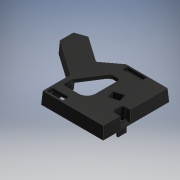
# Autodesk Inventor part: black_plastic_cover
Saved by Autodesk Inventor 2018 (Build 220112000, 112)
## iProperties
Created: 2019-03-10
Part Number: black_plastic_cover
Material: Generic
Document SubType Name: Modeling
Designer: ZEUSLAP
Density: 1 g/cm^3
Appearance: Default
Author: ZEUSLAP
Autodesk Inventor part; units mm, degrees
ref_plane "YZ Plane" through (0, 0, 0) normal (1, 0, 0) x (0, 1, 0)
ref_plane "XZ Plane" through (0, 0, 0) normal (0, 1, 0) x (-1, 0, 0)
ref_plane "XY Plane" through (0, 0, 0) normal (0, 0, 1) x (1, 0, 0)
sketch "Sketch1" plane through (0, 0, 0) normal (0, 0, 1) x (1, 0, 0)
  line L0 (18.3537, -19.4997) -> (-18.1463, -19.4997)
  line L1 (-18.2567, 19.3967) -> (18.3537, -19.4997) construction
  line L2 (18.1463, 19.4997) -> (-18.1463, -19.4997) construction
  line L3 (18.1463, 19.4997) -> (-6.8537, 19.4997) construction
  line L4 (-18.1463, -19.4997) -> (-18.1463, -2.9997) construction
  line L5 (18.1463, 19.4997) -> (-16.8537, 19.4997) construction
  line L6 (-16.8537, 19.4997) -> (-16.8537, 11.9997) construction
  line L7 (-6.8537, 19.4997) -> (-16.8537, 11.9997)
  line L8 (-38.8537, 19.4997) -> (-32.3537, 19.4997) construction
  line L9 (-16.8537, 11.9997) -> (-31.3344, 22.1392)
  line L10 (-31.3344, 22.1392) -> (-38.8537, 19.4997)
  line L11 (-38.8537, 19.4997) -> (-38.8537, 11.4997)
  line L12 (-38.8537, 11.4997) -> (-18.1463, -2.9997)
  line L13 (-18.1463, -19.4997) -> (-18.1463, -2.9997)
  line L14 (18.1463, 19.4997) -> (-6.8537, 19.4997) construction
  line L15 (-16.8537, 19.4997) -> (-38.8537, 19.4997) construction
  line L16 (-6.8537, 19.4997) -> (18.1463, 19.4997)
  line L17 (18.3537, -19.4997) -> (18.3537, -8.4997) construction
  line L18 (18.3537, -8.4997) -> (12.8537, -8.4997)
  line L19 (12.8537, -8.4997) -> (12.8537, -3.504)
  line L20 (12.8537, -3.504) -> (18.1463, -3.504)
  line L21 (18.1463, 19.4997) -> (18.1463, -3.504)
  line L22 (18.3537, -8.4997) -> (18.3537, -19.4997)
  line L23 (142.3108, -44.8623) -> (125.3108, -44.8623)
  line L24 (125.3108, -44.8623) -> (117.2807, -56.3304)
  line L25 (142.3108, -44.8623) -> (129.6921, -62.8836)
  line L26 (0, 0) -> (22, 0) construction
  line L27 (129.6921, -62.8836) -> (121.1921, -62.8836)
  line L28 (121.1921, -62.8836) -> (117.2807, -56.3304)
  line L29 (0, 84.0063) -> (0, -99.2035) construction
  dimension "d0" = 36.5
  dimension "d1" = 39
  dimension "d2" = 25
  dimension "d3" = 16.5
  dimension "d4" = 35
  dimension "d6" = 57
  dimension "d9" = 8
  dimension "d10" = 7.5
  dimension "d11" = 11
  dimension "d12" = 5
  dimension "d13" = 5.5
  dimension "d96" = 17
  dimension "d97" = 14
  dimension "d98" = 125
  dimension "d99" = 22
  dimension "d100" = 125
  dimension "d101" = 8.5
  dimension "d102" = 125
  dimension "d103" = 125
  constraints: 60 end point, 8 perpendicular, 5 horizontal, 3 parallel, 3 point on line, 1 equal length, 1 midpoint, 1 vertical
  measures "d0" distance of L0.start L0.end
  measures "d1" distance of L2.start L0.start
  measures "d2" distance of L2.start L3.end
  measures "d3" distance of L0.end L4.end
  measures "d4" distance of L2.start L5.end
  measures "d6" distance of L2.start L8.start
  measures "d9" distance of L8.start L11.end
  measures "d10" distance from line of L6.end L3
  measures "d11" distance of L0.start L17.end
  measures "d12" distance of L17.end L20.end
  measures "d13" distance of L17.end L18.end
  measures "d96" distance of L23.start L23.end
  measures "d97" distance of L23.end L24.end
  measures "d98" angle of L24 L23
  measures "d99" distance of L23.start L25.end
  measures "d100" angle of L25 L26
  measures "d101" distance of L25.end L27.end
  measures "d102" angle of L29 L12
  measures "d103" angle of L29 L9
extrude "Extrusion1" add sketch "Sketch1" along normal blind 7 contours L0 L13 L12 L11 L10 L9 L7 L16 L21 L20 L19 L18 L22
draft "FaceDraft1" angle 4 pull direction (0, 0, 1) fixed plane through (8.0488, 11.8318, 0) normal (0, 0, -1) faces at (1.4797, 19.4997, 2.3333)
draft "FaceDraft2" angle 4 pull direction (0, 0, 1) fixed plane through (8.0488, 11.8318, 0) normal (0, 0, -1) faces at (6.187, -19.4997, 4.6667)
draft "FaceDraft3" angle 4 pull direction (0, 0, 1) fixed plane through (8.0488, 11.8318, 0) normal (0, 0, -1) faces at (18.1463, 11.6686, 2.3333)
draft "FaceDraft4" angle 4 pull direction (0, 0, 1) fixed plane through (8.0488, 11.8318, 0) normal (0, 0, -1) faces at (18.3537, -15.6699, 2.3333)
draft "FaceDraft5" angle 4 pull direction (0, 0, 1) fixed plane through (8.0488, 11.8318, 0) normal (0, 0, -1) faces at (-18.1463, -13.8366, 2.3333)
draft "FaceDraft6" angle 4 pull direction (0, 0, 1) fixed plane through (8.0488, 11.8318, 0) normal (0, 0, -1) faces at (-38.8537, 14.1664, 2.3333)
draft "FaceDraft7" angle 4 pull direction (0, 0, 1) fixed plane through (8.0488, 11.8318, 0) normal (0, 0, -1) faces at (-24.7224, 1.6049, 4.6667)
draft "FaceDraft8" angle 4 pull direction (0, 0, 1) fixed plane through (8.0488, 11.8318, 0) normal (0, 0, -1) faces at (-26.5075, 18.7594, 2.3333)
draft "FaceDraft9" angle 4 pull direction (0, 0, 1) fixed plane through (8.0488, 11.8318, 0) normal (0, 0, -1) faces at (-10.4046, 16.8366, 2.3333)
draft "FaceDraft10" angle 5 pull direction (0, 0, 1) fixed plane through (8.0488, 11.8318, 0) normal (0, 0, -1) faces at (16.3572, -8.4997, 2.3333)
draft "FaceDraft11" angle 5 pull direction (0, 0, 1) fixed plane through (8.0488, 11.8318, 0) normal (0, 0, -1) faces at (16.2189, -3.504, 2.3333)
fillet "Fillet1" radius 2 2 edges at (12.8537, -3.1978, 3.5) (12.8537, -8.8059, 3.5)
fillet "Fillet2" radius 1 2 edges at (-17.9016, -2.8723, 3.5) (-16.8487, 11.6975, 3.5)
sketch "Sketch2" plane through (0, 0, 7) normal (0, 0, 1) x (1, 0, 0)
  line L0 (17.6568, -2.8916) -> (17.6568, 19.0102) construction
  line L1 (17.6568, 19.0102) -> (-5.3432, 19.0102) construction
  line L2 (17.6568, 19.0102) -> (6.1568, 19.0102) construction
  line L3 (17.6568, 19.0102) -> (-6.6905, 19.0102) construction
  line L4 (6.1568, 19.0102) -> (6.1568, 18.2602) construction
  line L5 (6.1568, 18.2602) -> (6.1568, 15.2602)
  line L6 (6.1568, 15.2602) -> (-5.3432, 15.2602)
  line L7 (-5.3432, 15.2602) -> (-5.3432, 18.2602)
  line L8 (-5.3432, 18.2602) -> (6.1568, 18.2602)
  line L9 (-17.6568, -19.0102) -> (17.8642, -19.0102) construction
  line L10 (-17.6568, -19.0102) -> (-16.6568, -19.0102) construction
  line L11 (-16.6568, -19.0102) -> (-16.6568, -18.0102) construction
  line L12 (-16.6568, -18.0102) -> (-6.9068, -18.0102)
  line L13 (-6.9068, -18.0102) -> (-6.9068, -14.5102)
  line L14 (-6.9068, -14.5102) -> (-16.6568, -14.5102)
  line L15 (-16.6568, -14.5102) -> (-16.6568, -18.0102)
  line L16 (-17.6568, -3.2642) -> (-17.6568, -19.0102) construction
  line L17 (-17.6568, -19.0102) -> (-15.1568, -19.0102) construction
  line L18 (-15.1568, -19.0102) -> (-15.1568, -10.0102) construction
  line L19 (-14.1568, -10.0102) -> (-5.6568, -10.0102) construction
  line L20 (-0.6568, -5.0102) -> (-0.6568, 8.4898)
  line L21 (-14.1568, -10.0102) -> (-5.6568, -10.0102)
  line L22 (-1.6568, 9.4898) -> (-5.6109, 9.4898)
  line L23 (-15.1568, -9.0102) -> (-15.1568, -4.8039)
  line L24 (-14.998, -4.2632) -> (-6.4521, 9.0305)
  arc A0 (-5.6568, -10.0102) -> (-0.6568, -5.0102) centre (-5.6568, -5.0102) ccw
  arc A1 (-0.6568, 8.4898) -> (-1.6568, 9.4898) centre (-1.6568, 8.4898) ccw
  arc A2 (-15.1568, -9.0102) -> (-14.1568, -10.0102) centre (-14.1568, -9.0102) ccw
  arc A3 (-14.998, -4.2632) -> (-15.1568, -4.8039) centre (-14.1568, -4.8039) ccw
  arc A4 (-5.6109, 9.4898) -> (-6.4521, 9.0305) centre (-5.6109, 8.4898) ccw
  line L25 (17.6568, 19.0102) -> (8.6568, 19.0102) construction
  line L26 (17.6568, 19.0102) -> (11.6568, 19.0102) construction
  point P0 (0, 0)
  point P1 (-0.6568, -10.0102)
  point P2 (-0.6568, 9.4898)
  point P3 (-6.1568, 9.4898)
  point P4 (-15.1568, -4.5102)
  dimension "d29" = 23
  dimension "d30" = 11.5
  dimension "d31" = 0.75
  dimension "d32" = 3
  dimension "d33" = 1
  dimension "d34" = 1
  dimension "d35" = 9.75
  dimension "d36" = 3.5
  dimension "d37" = 2.5
  dimension "d38" = 9
  dimension "d40" = 19.5
  dimension "d41" = 5.5
  dimension "d42" = 5.5
  dimension "d46" = 5
  dimension "d47" = 1
  constraints: 46 end point, 17 point on line, 12 perpendicular, 10 point on circle, 10 tangent, 5 centre point, 3 equal radius, 2 horizontal, 1 parallel, 1 vertical
  measures "d29" distance of L0.end L1.end
  measures "d30" distance of L0.end L2.end
  measures "d31" distance of L2.end L4.end
  measures "d32" distance of L4.end L5.end
  measures "d33" distance of L9.start L10.end
  measures "d34" distance of L10.end L11.end
  measures "d35" distance of L11.end L12.end
  measures "d36" distance of L12.end L13.end
  measures "d37" distance of L9.start L17.end
  measures "d38" distance of L17.end L18.end
  measures "d40" distance of point (-0.657, -10.01) point (-0.657, 9.49)
  measures "d41" distance of point (-0.657, 9.49) point (-6.157, 9.49)
  measures "d42" distance of L18.end point (-15.157, -4.51)
  measures "d46" radius of A0
  measures "d47" radius of A1
shell "Shell1" thickness 2 removed faces 1 at (8.4128, 11.7589, 0)
extrude "Extrusion2" cut sketch "Sketch2" against normal up to surface (2 mm away) from surface at 0
sketch "Sketch4" plane through (0, 0, 7) normal (0, 0, 1) x (1, 0, 0)
  line L0 (17.7605, -2.8876) -> (17.7605, 19.0105) construction
  line L1 (17.7605, 19.0105) -> (6.2605, 19.0105) construction
  line L2 (-17.7605, -19.0105) -> (17.7605, -19.0105) construction
  line L3 (17.7605, 19.0105) -> (8.7605, 19.0105) construction
  line L4 (8.7605, 19.0105) -> (8.7605, 3.0105) construction
  line L5 (17.7605, 19.0105) -> (11.7605, 19.0105) construction
  line L6 (11.7605, 19.0105) -> (11.7605, -1.4895) construction
  line L7 (8.7605, 3.0105) -> (10.1193, -1.4895)
  line L8 (10.1193, -1.4895) -> (4.3754, -3.2238)
  line L9 (4.3754, -3.2238) -> (3.0166, 1.2762)
  line L10 (3.0166, 1.2762) -> (8.7605, 3.0105)
  dimension "d68" = 9
  dimension "d69" = 16
  dimension "d70" = 6
  dimension "d71" = 20.5
  dimension "d72" = 6
  constraints: 22 end point, 4 perpendicular, 1 point on line
  measures "d68" distance of L0.end L3.end
  measures "d69" distance of L3.end L4.end
  measures "d70" distance of L0.end L5.end
  measures "d71" distance of L5.end L6.end
  measures "d72" distance of L7.end L8.end
extrude "Extrusion3" cut sketch "Sketch4" against normal up to surface (2 mm away)
sketch "Sketch6" plane through (0, 0, 7) normal (0, 0, 1) x (1, 0, 0)
  line L0 (4.3754, -3.2238) -> (3.0166, 1.2762) projected
  line L1 (3.0166, 1.2762) -> (8.7582, 3.0098)
  line L2 (8.7582, 3.0098) -> (10.1169, -1.4902)
  line L3 (10.1169, -1.4902) -> (4.3754, -3.2238)
  line L4 (4.3754, -3.2238) -> (3.0166, 1.2762)
  line L5 (3.0166, 1.2762) -> (2.7276, 2.2335) construction
  line L6 (3.0166, 1.2762) -> (2.0593, 0.9871) construction
  line L7 (2.7276, 2.2335) -> (1.7803, 1.9475)
  line L8 (10.1193, -1.4895) -> (4.3754, -3.2238) construction
  line L9 (3.0166, 1.2762) -> (10.1193, -1.4895) construction
  line L10 (8.7582, 3.0098) -> (4.3754, -3.2238) construction
  line L11 (1.7803, 1.9475) -> (3.5898, -4.3411)
  line L12 (3.5898, -4.3411) -> (11.5393, -2.0538)
  line L13 (11.5393, -2.0538) -> (9.6034, 4.2119)
  line L14 (9.6034, 4.2119) -> (2.7276, 2.2335)
  point P0 (0, 0)
  dimension "d75" = 1
  dimension "d76" = 1
  constraints: 26 end point, 7 perpendicular, 3 point on line
  measures "d75" distance of L0.end L5.end
  measures "d76" distance of L0.end L6.end
extrude "Extrusion4" add sketch "Sketch6" against normal blind 4
sketch "Sketch7" plane through (0, 0, 3) normal (0, 0, -1) x (-1, 0, 0)
  point P0 (0, 0)
sketch "Sketch8" plane through (0, 0, 3) normal (0, 0, -1) x (-1, 0, 0)
  point P0 (0, 0)
sketch "Sketch9" plane through (1.7803, 1.9475, 3) normal (-0.9610086, -0.2765185, 0) x (0, 0, 1)
  line L0 (2, 0) -> (0, 0) construction
  line L1 (2, 0) -> (2, -6.5438) construction
  line L2 (0, 0) -> (2, -6.5438) construction
  line L3 (2, -6.5438) -> (0, -6.5438) construction
  line L4 (2, 0) -> (0, -6.5438) construction
  line L5 (1, -3.2719) -> (-9, -3.2719) construction
  arc A0 (0, -6.5438) -> (0, 0) centre (-9, -3.2719) ccw
  arc A1 (-0.6158, -6.5438) -> (-0.6209, 0.0129) centre (-9, -3.2719) ccw
  line L6 (0, 0) -> (-0.6209, 0.0129)
  line L7 (0, -6.5438) -> (-0.6158, -6.5438)
  point P0 (-3, -1.3793)
  point P1 (0, 0.0129)
  constraints: 10 end point, 4 point on circle, 2 centre point, 2 coincident, 2 horizontal, 1 midpoint
extrude "Extrusion5" add sketch "Sketch9" against normal blind 8
sketch "Sketch10" plane through (0, 0, 0) normal (0, 0, -1) x (-1, 0, 0)
  line L0 (-18.1463, -3.504) -> (-17.6568, -2.8916) projected
  line L1 (-14.8537, -8.4997) -> (-18.3537, -8.4997) projected
  line L2 (-18.1463, -3.504) -> (-15.1463, -3.504)
  line L3 (-15.1463, -3.504) -> (-15.1463, -8.4997)
  line L4 (-15.1463, -8.4997) -> (-18.1463, -8.4997)
  line L5 (-18.1463, -8.4997) -> (-18.1463, -3.504)
  point P0 (0, 0)
  dimension "d82" = 3
  constraints: 8 end point, 2 parallel, 1 horizontal, 1 perpendicular, 1 point on line
  measures "d82" distance of L3.end L4.end
extrude "Extrusion6" add sketch "Sketch10" against normal blind 0.75
sketch "Sketch11" plane through (0, 0, 0.75) normal (0, 0, 1) x (1, 0, 0)
  line L0 (15.1463, -3.504) -> (14.8537, -3.504) projected
  line L1 (15.1463, -3.504) -> (15.1463, -9.8859)
  line L2 (15.1463, -9.8859) -> (16.1463, -9.8859)
  line L3 (16.1463, -9.8859) -> (16.1463, -2.5236)
  line L4 (16.1463, -2.5236) -> (15.1463, -2.5236)
  line L5 (15.1463, -2.5236) -> (15.1463, -3.504)
  point P0 (0, 0)
  dimension "d85" = 1
  constraints: 10 end point, 4 perpendicular, 1 point on line, 1 vertical
  measures "d85" distance of L1.end L2.end
extrude "Extrusion7" add sketch "Sketch11" along normal blind 0.5
sketch "Sketch12" plane through (0, 0, 0) normal (0, 0, -1) x (-1, 0, 0)
  line L0 (-16.1463, -3.504) -> (-16.1463, -8.4997) projected
  line L1 (-16.1463, -3.504) -> (-16.1463, -8.4997)
  line L2 (-15.1463, -8.4997) -> (-18.1463, -8.4997) projected
  line L3 (-16.1463, -8.4997) -> (-15.1463, -8.4997)
  line L4 (-15.1463, -8.4997) -> (-15.1463, -3.504)
  line L5 (-15.1463, -3.504) -> (-16.1463, -3.504)
  point P0 (0, 0)
  point P1 (-18.25, -8.5)
  constraints: 8 end point, 3 perpendicular, 1 vertical, 1 other
extrude "Extrusion8" add sketch "Sketch12" along normal blind 5
sketch "Sketch13" plane through (16.1463, -8.4997, 0) normal (1, 0, 0) x (0, 0, -1)
  line L0 (0, 4.9957) -> (5, 4.9957) construction
  line L1 (0, 4.9957) -> (0, 2.4978) construction
  line L2 (0, 0) -> (0, 4.9957) construction
  line L3 (0, 4.9957) -> (0, 3) construction
  line L4 (0, 3) -> (4.5, 3)
  line L5 (4.5, 3) -> (4.5, 2.0076)
  line L6 (0, 2.0076) -> (-5, 1.5702) projected
  line L7 (4.5, 2.0076) -> (0, 2.0076)
  line L8 (0, 2.0076) -> (0, 3)
  point P0 (0, 8.4997)
  dimension "d90" = 1.9957
  dimension "d91" = 4.5
  dimension "d92" = 0.9924
  constraints: 12 end point, 4 perpendicular, 1 midpoint, 1 point on line
  measures "d90" distance of L0.start L3.end
  measures "d91" distance of L3.end L4.end
  measures "d92" distance of L4.end L5.end
extrude "Extrusion9" add sketch "Sketch13" along normal blind 1.5
draft "FaceDraft12" angle 15 pull direction (0, 0, -1) fixed plane through (17.313, -7.8305, 0) normal (0, 0, -1) faces at (17.6463, -6.1613, -3)
body "Solid1"
